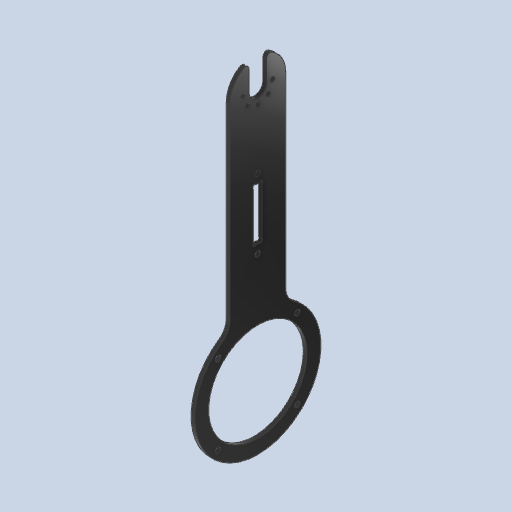
# Autodesk Inventor part: ForeArm_outside_frame
Saved by Autodesk Inventor 2022.3 (Build 263350000, 350)
## iProperties
Part Number: ForeArm_outside_frame
Material: GFRP
Document SubType Name: Modeling
Designer: Masato Kubotera
Density: 1.75 g/cm^3
Appearance: 低 光沢 - 黒
Description: GFRP T2
Mass: 17.9898 g
Surface Area: 119.841 cm^2
Volume: 10.2799 cm^3
Author: Masato Kubotera
Revision Number: Rev.1 Specifications for RoboCup 2022
Autodesk Inventor part; units mm, degrees
ref_plane "YZ Plane" through (0, 0, 0) normal (1, 0, 0) x (0, 1, 0)
ref_plane "XZ Plane" through (0, 0, 0) normal (0, 1, 0) x (-1, 0, 0)
ref_plane "XY Plane" through (0, 0, 0) normal (0, 0, 1) x (1, 0, 0)
sketch "スケッチ1" plane through (0, 0, 0) normal (0, 1, 0) x (-1, 0, 0)
  circle A0 centre (0, 0) radius 5.05
  line L0 (-8.5, 0) -> (8.5, 0) construction
  circle A1 centre (-8.5, 0) radius 1.35
  circle A2 centre (-6.0104, -6.0104) radius 1.35
  circle A3 centre (0, -8.5) radius 1.35
  circle A4 centre (6.0104, -6.0104) radius 1.35
  circle A5 centre (0, -145.8097) radius 16 construction
  line L1 (0, 0) -> (0, -145.8097) construction
  arc A6 (-20.3699, -115.9088) -> (20.3699, -115.9088) centre (0, -145.8097) ccw
  circle A7 centre (-8.5, 0) radius 2.4 construction
  line L2 (-16, 31) -> (16, 31) construction
  line L3 (16, 31) -> (16, -12) construction
  line L4 (16, -12) -> (-16, -12) construction
  line L5 (-16, -12) -> (-16, 31) construction
  line L6 (-16, 31) -> (16, -12) construction
  line L7 (16, 31) -> (-16, -12) construction
  arc A8 (-16, 0) -> (-10.583, -12) centre (0, 0) ccw construction
  arc A9 (10.583, -12) -> (16, 0) centre (0, 0) ccw construction
  line L8 (-16, -107.6443) -> (-16, 0)
  line L9 (16, -107.6443) -> (16, 0)
  circle A10 centre (0, -82.5) radius 1.6
  line L10 (0, -145.8097) -> (-25.5832, -120.2265) construction
  circle A11 centre (-22.7548, -123.055) radius 4 construction
  circle A12 centre (-22.7548, -123.055) radius 1.6
  circle A13 centre (-22.7548, -168.5645) radius 1.6
  circle A14 centre (22.7548, -168.5645) radius 1.6
  circle A15 centre (22.7548, -123.055) radius 1.6
  line L11 (30.6064, -21.0119) -> (2.8936, -37.0119) construction
  line L12 (2.8936, -37.0119) -> (-18.6064, 0.2272) construction
  line L13 (-18.6064, 0.2272) -> (9.1064, 16.2272) construction
  line L14 (9.1064, 16.2272) -> (30.6064, -21.0119) construction
  line L15 (30.6064, -21.0119) -> (-18.6064, 0.2272) construction
  line L16 (2.8936, -37.0119) -> (9.1064, 16.2272) construction
  line L17 (16.75, -29.0119) -> (-4.75, 8.2272) construction
  circle A16 centre (0, -42.5) radius 1.6
  line L18 (-2.5, -47.5) -> (2.5, -47.5) construction
  line L19 (2.5, -47.5) -> (2.5, -57.5) construction
  line L20 (2.5, -57.5) -> (-2.5, -57.5) construction
  line L21 (-2.5, -57.5) -> (-2.5, -47.5) construction
  line L22 (-2.5, -47.5) -> (2.5, -57.5) construction
  line L23 (2.5, -47.5) -> (-2.5, -57.5) construction
  line L24 (-2.5, -52.5) -> (2.5, -52.5) construction
  circle A17 centre (0, -62.5) radius 1.6
  line L25 (2.8936, -37.0119) -> (49.2811, -117.3573) construction
  line L26 (0, -145.8097) -> (49.2811, -117.3573) construction
  line L27 (-2.5, -47.5) -> (2.5, -47.5) construction
  line L28 (2.5, -47.5) -> (2.5, -77.5) construction
  line L29 (2.5, -77.5) -> (-2.5, -77.5) construction
  line L30 (-2.5, -77.5) -> (-2.5, -47.5) construction
  line L31 (-2.5, -47.5) -> (2.5, -77.5) construction
  line L32 (2.5, -47.5) -> (-2.5, -77.5) construction
  line L33 (-2.55, -47.45) -> (2.55, -47.45)
  line L34 (2.55, -47.45) -> (2.55, -77.55)
  line L35 (2.55, -77.55) -> (-2.55, -77.55)
  line L36 (-2.55, -77.55) -> (-2.55, -47.45)
  line L37 (-2.55, -47.45) -> (2.55, -77.55) construction
  line L38 (2.55, -47.45) -> (-2.55, -77.55) construction
  arc A18 (-1.0651, -47.45) -> (-2.55, -48.9349) centre (-1.8075, -48.1925) ccw
  arc A19 (2.55, -48.9349) -> (1.0651, -47.45) centre (1.8075, -48.1925) ccw
  line L39 (-2.5, -62.5) -> (2.5, -62.5) construction
  arc A20 (-2.55, -76.0651) -> (-1.0651, -77.55) centre (-1.8075, -76.8075) ccw
  arc A21 (1.0651, -77.55) -> (2.55, -76.0651) centre (1.8075, -76.8075) ccw
  arc A22 (16, 0) -> (8.0571, 13.8233) centre (0, 0) ccw
  circle A23 centre (0, -145.8097) radius 28.1801
  line L40 (-5.05, 0) -> (-5.05, 12.0954)
  line L41 (5.05, 0) -> (5.05, 12.0954)
  circle A24 centre (8.5, 0) radius 1.35
  arc A25 (-8.0571, 13.8233) -> (-16, 0) centre (0, 0) ccw
  arc A26 (-5.05, 12.0954) -> (-8.0571, 13.8233) centre (-7.05, 12.0954) ccw
  arc A27 (8.0571, 13.8233) -> (5.05, 12.0954) centre (7.05, 12.0954) ccw
  arc A28 (-20.3699, -115.9088) -> (-16, -107.6443) centre (-26, -107.6443) ccw
  arc A29 (16, -107.6443) -> (20.3699, -115.9088) centre (26, -107.6443) ccw
  point P0 (0, 9.5)
  point P1 (0, 9.5)
  point P2 (-16, -113.3598)
  point P3 (16, -113.3598)
  point P4 (6, -10.3923)
  point P5 (0, -52.5)
  point P6 (0, -62.5)
  point P7 (1.0651, -77.55)
  point P8 (-1.0651, -77.55)
  point P9 (-2.55, -76.0651)
  point P10 (2.55, -48.9349)
  point P11 (2.55, -76.0651)
  point P12 (0, -181.9899)
  point P13 (-5.05, 15.1821)
  point P14 (5.05, 15.1821)
  point P15 (5.05, 9.6596)
  point P16 (5.05, 0)
  dimension "d0" = 10.1
  dimension "d1" = 17
  dimension "d2" = 2.7
  dimension "d5" = 180
  dimension "d7" = 32
  dimension "d8" = 145.8098
  dimension "d9" = 72.3602
  dimension "d10" = 4.8
  dimension "d11" = 32
  dimension "d12" = 43
  dimension "d14" = 9.5
  dimension "d17" = 3.2
  dimension "d23" = 32
  dimension "d24" = 45
  dimension "d25" = 8
  dimension "d26" = 3.2
  dimension "d29" = 360
  dimension "d33" = 32
  dimension "d34" = 43
  dimension "d36" = 9.5
  dimension "d37" = 150
  dimension "d38" = 3.2
  dimension "d40" = 5
  dimension "d41" = 10
  dimension "d42" = 40
  dimension "d43" = 20
  dimension "d44" = 42.5
  dimension "d45" = 30
  dimension "d46" = 1.05
  dimension "d47" = 0.05
  dimension "d48" = 0.05
  dimension "d49" = 16
  dimension "d50" = 181.9898
  dimension "d53" = 90
  dimension "d54" = 2
  dimension "d55" = 10
  constraints: 85 end point, 34 point on circle, 29 centre point, 18 midpoint, 16 point on line, 16 symmetric about line, 13 tangent, 10 coincident, 10 parallel, 6 perpendicular, 4 horizontal, 3 collinear, 2 equal radius, 2 vertical, 26 other
  measures "d1" distance of L0.start L0.end
  measures "d2" diameter of A1
  measures "d7" diameter of A5
  measures "d8" distance of L1.end point (0, 0)
  measures "d9" diameter of A6
  measures "d10" diameter of A7
  measures "d11" distance of L3.end L4.end
  measures "d12" distance of L2.end L3.end
  measures "d14" distance of point (0, 0) point (0, 9.5)
  measures "d17" diameter of A10
  measures "d23" distance of point (16, -113.36) point (-16, -113.36)
  measures "d24" angle of L10 L1
  measures "d25" diameter of A11
  measures "d26" diameter of A12
  measures "d33" distance of L12.end L13.end
  measures "d34" distance of L11.end L12.end
  measures "d36" distance of L17.end point (0, 0)
  measures "d37" angle of L1 L12
  measures "d38" diameter of A16
  measures "d40" distance of L19.end L20.end
  measures "d41" distance of L18.end L19.end
  measures "d42" distance of A10.centre A16.centre
  measures "d43" distance of A17.centre A16.centre
  measures "d44" distance of A16.centre point (0, 0)
  measures "d45" distance of L27.end L28.end
  measures "d46" radius of A18
  measures "d47" distance between parallel lines of L33 L27
  measures "d48" distance between parallel lines of L36 L30
  measures "d49" radius of A22
  measures "d50" distance of point (0, -181.99) point (0, 0)
  measures "d53" angle of L0 L1
  measures "d54" radius of A26
  measures "d55" radius of A28
extrude "押し出し1" add sketch "スケッチ1" along normal blind 2 contours L41 A27 A22 L9 A29 A6 A28 L8 A25 A26 L40 A0
equation "\"d36\" = d14"
